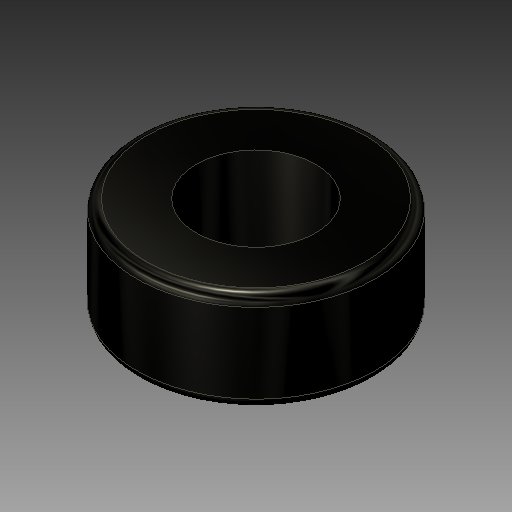
# Autodesk Inventor part: セットカラー 内径6 外径12 幅5
Saved by Autodesk Inventor 2017.3 (Build 213256000, 256)
## iProperties
Part Number: セットカラー 内径6 外径12 幅5
Material: アルミニウム 6061
Document SubType Name: Modeling
Designer: user
Density: 2.7 g/cm^3
Appearance: ガンメタル
Mass: 1.13439 g
Surface Area: 4.35986 cm^2
Volume: 0.420145 cm^3
Author: user
Autodesk Inventor part; units mm, degrees
ref_plane "YZ Plane" through (0, 0, 0) normal (1, 0, 0) x (0, 1, 0)
ref_plane "XZ Plane" through (0, 0, 0) normal (0, 1, 0) x (-1, 0, 0)
ref_plane "XY Plane" through (0, 0, 0) normal (0, 0, 1) x (1, 0, 0)
sketch "スケッチ1" plane through (0, 0, 0) normal (0, 1, 0) x (-1, 0, 0)
  circle A0 centre (0, 0) radius 3
  circle A1 centre (0, 0) radius 6
  dimension "d0" = 6
  dimension "d1" = 12
  constraints: 2 centre point, 2 coincident
  measures "d0" diameter of A0
  measures "d1" diameter of A1
extrude "押し出し1" add sketch "スケッチ1" along normal blind 5
fillet "フィレット1" radius 0.5 1 edges at (6, 5, 0)
fillet "フィレット2" radius 0.5 1 edges at (6, 0, 0)
